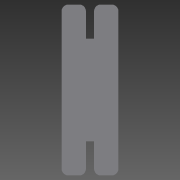
# Autodesk Inventor part: straight
Saved by Autodesk Inventor 2015 (Build 190159000, 159)
## iProperties
Created: 2015-02-16
Part Number: straight
Material: Generic
Document SubType Name: Modeling
Designer: Iain
Density: 1 g/cm^3
Appearance: Default
Author: Iain
Autodesk Inventor part; units mm, degrees
ref_plane "YZ Plane" through (0, 0, 0) normal (1, 0, 0) x (0, 1, 0)
derived "hex.ipt"
sketch "Sketch1" plane through (0, 0, 0) normal (0, 1, 0) x (-1, 0, 0)
  line L0 (8.3333, 25) -> (-8.3333, 25)
  line L1 (-8.3333, 25) -> (-8.3333, -25)
  line L2 (-8.3333, -25) -> (8.3333, -25)
  line L3 (8.3333, -25) -> (8.3333, 25)
  point P0 (0, 0)
  point P1 (0, -25)
  point P2 (-8.3333, 0)
  dimension "d1" = 16.6667
  dimension "strightLength" = 50
  constraints: 8 end point, 2 midpoint, 2 parallel, 1 horizontal, 1 horizontal alignment, 1 perpendicular, 1 vertical alignment
  measures "d1" distance of L0.start L0.end
  measures "strightLength" distance of L2.end L0.start
extrude "Extrusion1" add sketch "Sketch1" along normal blind 2.5
sketch "Sketch2" plane through (0, 2.5, 0) normal (0, 1, 0) x (1, 0, 0)
  line L0 (-8.3333, -25) -> (8.3333, -25) projected
  line L1 (-1.175, -25) -> (1.175, -25)
  line L2 (1.175, -25) -> (1.175, -15)
  line L3 (1.175, -15) -> (-1.175, -15)
  line L4 (-1.175, -15) -> (-1.175, -25)
  point P0 (0, 0)
  point P1 (0, -15)
  point P2 (0, -25)
  point P3 (0, -25)
  point P4 (0, -25)
  dimension "d5" = 2.35
  dimension "d6" = 10
  constraints: 8 end point, 4 midpoint, 2 parallel, 1 coincident, 1 horizontal, 1 perpendicular, 1 vertical alignment
  measures "d5" distance of L2.end L3.end
  measures "d6" distance of L1.end L2.end
extrude "Extrusion2" cut sketch "Sketch2" against normal through all
sketch "Sketch3" plane through (0, 2.5, 0) normal (0, 1, 0) x (1, 0, 0)
  line L0 (1.175, -15) -> (1.175, -25) projected
  arc A0 (1.175, -18.75) -> (1.175, -21.25) centre (32.4125, -20) ccw
  line L1 (1.15, -19.1491) -> (1.15, -21.371) construction
  line L2 (1.175, -21.25) -> (1.175, -18.75)
  point P0 (0, 0)
  point P1 (1.175, -20)
  point P2 (1.175, -20)
  point P3 (1.175, -20)
  point P4 (1.175, -20)
  dimension "d9" = 2.5
  dimension "d10" = 0.025
  constraints: 4 end point, 4 midpoint, 2 point on circle, 2 vertical alignment, 1 centre point, 1 horizontal alignment, 1 tangent, 1 vertical
  measures "d9" distance of L2.start L2.end
  measures "d10" distance from line of L1 point (1.175, -20)
extrude "Extrusion3" add sketch "Sketch3" against normal blind 2.5
ref_plane "Work Plane1" through (0, 2.5, 25) normal (1, 0, 0) x (0, 0, -1)
mirror "Mirror1" about plane through (0, 2.5, 25) normal (1, 0, 0) of "Extrusion3"
ref_plane "Work Plane2" through (8.3333, 0, 0) normal (0, 0, 1) x (1, 0, 0)
mirror "Mirror2" about plane through (8.3333, 0, 0) normal (0, 0, 1) of "Extrusion3", "Mirror1", "Extrusion2"
fillet "slotFillet" radius 2 4 edges at (-1.175, 1.25, -25) (1.175, 1.25, -25) (-1.175, 1.25, 25) (1.175, 1.25, 25)
fillet "edgeFillet" radius 2 4 edges at (-8.3333, 1.25, 25) (8.3333, 1.25, 25) (8.3333, 1.25, -25) (-8.3333, 1.25, -25)
equation "\"d1\" = 0.333333 * hexWidth"
equation "\"strightLength\" = hexWidth"
equation "\"d3\" = materialThickness"
equation "\"d5\" = slotWidth"
equation "\"d6\" = slotDepth"
equation "\"d7\" = materialThickness"
equation "\"d9\" = 0.25 * slotDepth"
equation "\"d10\" = slotNoduleHeight"
equation "\"d13\" = materialThickness"
equation "\"hexWidth\" = 50"
equation "\"materialThickness\" = 2.5"
equation "\"slotWidth\" = 2.35"
equation "\"slotDepth\" = 10"
equation "\"slotNoduleHeight\" = 0.025"
body "Solid1"
